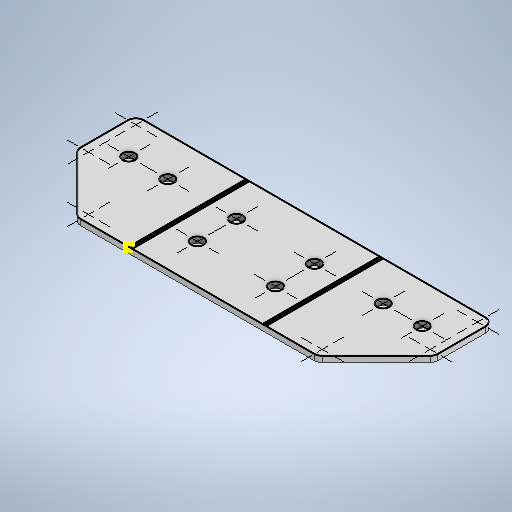
# Autodesk Inventor part: Head1
Saved by Autodesk Inventor 2026.1 (Build 301233000, 233)
## iProperties
Created: 2025-08-16
Part Number: Head1
Material: Generic
Document SubType Name: Modeling
Designer: chris
Density: 1 g/cm^3
Appearance: Default
Author: chris
Autodesk Inventor part; units mm, degrees
ref_plane "YZ Plane" through (0, 0, 0) normal (1, 0, 0) x (0, 1, 0)
ref_plane "XZ Plane" through (0, 0, 0) normal (0, 1, 0) x (-1, 0, 0)
ref_plane "XY Plane" through (0, 0, 0) normal (0, 0, 1) x (1, 0, 0)
sketch "Sketch1" plane through (0, 0, 0) normal (0, 1, 0) x (-1, 0, 0)
  line L0 (-0.4496, -30) -> (-0.4496, 0)
  line L1 (-34.7289, 0) -> (-34.7289, -30)
  circle A0 centre (-45.1786, -20) radius 1.55
  circle A1 centre (10, -20) radius 1.55
  circle A2 centre (-55.1786, -20) radius 1.55
  circle A3 centre (20, -20) radius 1.55
  circle A4 centre (-27.5893, -10) radius 1.55
  circle A5 centre (-27.5893, -20) radius 1.55
  circle A6 centre (-7.5893, -10) radius 1.55
  circle A7 centre (-7.5893, -20) radius 1.55
  arc A8 (13.7758, -0.5858) -> (12.3616, 0) centre (12.3616, -2) ccw
  line L2 (27.6042, -14.4142) -> (13.7758, -0.5858)
  arc A9 (28.19, -15.8284) -> (27.6042, -14.4142) centre (26.19, -15.8284) ccw
  line L3 (28.19, -15.8284) -> (28.19, -28)
  arc A10 (26.19, -30) -> (28.19, -28) centre (26.19, -28) ccw
  arc A11 (-47.5401, 0) -> (-48.9543, -0.5858) centre (-47.5401, -2) ccw
  line L4 (-48.9543, -0.5858) -> (-62.7828, -14.4142)
  arc A12 (-62.7828, -14.4142) -> (-63.3686, -15.8284) centre (-61.3686, -15.8284) ccw
  line L5 (-63.3686, -28) -> (-63.3686, -15.8284)
  arc A13 (-63.3686, -28) -> (-61.3686, -30) centre (-61.3686, -28) ccw
  line L6 (-47.5401, 0) -> (12.3616, 0)
  line L7 (26.19, -30) -> (-61.3686, -30)
  line L8 (-35.1786, -30) -> (-35.1786, 0)
  line L9 (-34.2793, 0) -> (-34.2793, -30)
  line L10 (-0.8993, -30) -> (-0.8993, 0)
  line L11 (0, 0) -> (0, -30)
  constraints: 24 end point, 14 centre point, 12 equal radius, 12 point on circle, 12 point on line, 12 tangent, 8 vertical, 7 parallel, 3 perpendicular, 2 horizontal, 55 other
extrude "Extrusion1" add sketch "Sketch1" against normal blind 1.5
body "Solid1"
